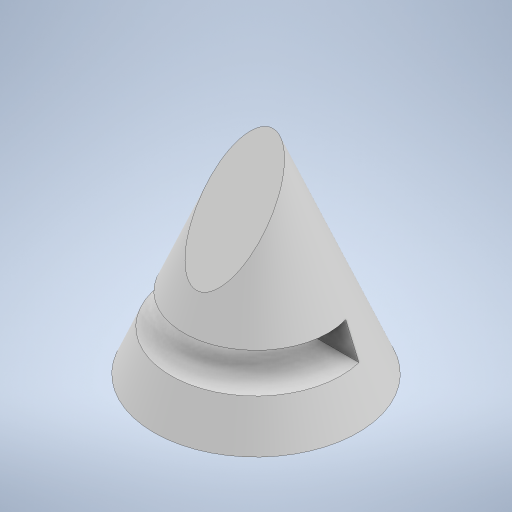
# Autodesk Inventor part: 20
Saved by Autodesk Inventor 2024 (Build 280153000, 153)
## iProperties
Created: 2023-11-17
Part Number: 20
Material: Типовые
Document SubType Name: Modeling
Designer: User
Density: 1 g/cm^3
Appearance: По умолчанию
Author: User
Autodesk Inventor part; units mm, degrees
ref_plane "YZ Plane" through (0, 0, 0) normal (1, 0, 0) x (0, 1, 0)
ref_plane "XZ Plane" through (0, 0, 0) normal (0, 1, 0) x (-1, 0, 0)
ref_plane "XY Plane" through (0, 0, 0) normal (0, 0, 1) x (1, 0, 0)
sketch "Эскиз1" plane through (0, 0, 0) normal (1, 0, 0) x (0, 1, 0)
  line L0 (0, 0) -> (120, 0)
  line L1 (120, 0) -> (0, -50)
  line L2 (0, -50) -> (0, 0)
  dimension "d0" = 50
  dimension "d1" = 120
  constraints: 6 end point, 1 horizontal, 1 perpendicular
  measures "d0" distance of L1.end L0.start
  measures "d1" distance of L0.start L0.end
revolve "Вращение1" add sketch "Эскиз1" angle 360 about axis through (0, 0, 0) along (0, 1, 0)
sketch "Эскиз3" plane through (0, 0, 0) normal (1, 0, 0) x (0, 1, 0)
  line L0 (100, 0) -> (100, -8.3333)
  line L1 (0, -50) -> (120, 0) projected
  line L2 (0, 50) -> (120, 0) projected
  line L3 (50, 29.1667) -> (50, 0)
  line L4 (0, 0) -> (20, 0)
  line L5 (20, 41.6667) -> (20, 0)
  line L6 (20, -10) -> (35, -10)
  line L7 (35, -10) -> (35, 35.4167)
  line L8 (0, -50) -> (0, 50) projected
  line L9 (100, -8.3333) -> (50, 29.1667)
  line L10 (20, 0) -> (20, -10)
  dimension "d8" = 100
  dimension "d10" = 15
  dimension "d11" = 20
  dimension "d12" = 50
  constraints: 16 end point, 5 point on line, 2 perpendicular, 1 horizontal, 1 vertical
  measures "d8" distance between parallel lines of L8 L0
  measures "d10" distance between parallel lines of L7 L5
  measures "d11" distance between parallel lines of L8 L5
  measures "d12" distance between parallel lines of L8 L3
extrude "Выдавливание2" cut sketch "Эскиз3" along normal mid plane 100 contours L9 L2 L1 | L5 L2 L7 L6 L10
